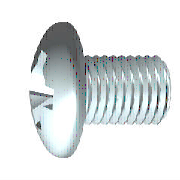
# Autodesk Inventor part: ISO 7045 - M4 x 6 - 4.8 - Z
Saved by Autodesk Inventor 2019.4 (Build 234330000, 330)
## iProperties
Created: 2018-01-05
Part Number: ISO 7045 - M4 x 6 - 4.8 - Z
Material: Stal
Description: Wkręt z łbem stożkowym ściętym z wgłębieniem krzyżowym w kształcie Z - Klasa dokładności A
Document SubType Name: Modeling
Standard: ISO 7045
Designer: barto
Standard Revision: Third edition 2011-09-01
Standards Organization: ISO
Language: pl-PL
Size Designation: M4 x 6 - 4.8 - Z
Categories: <MemberInstance><Categories><Category DisplayName="Mocowania" InternalName="e4da775c-781d-43d5-af7c-5136215cf5a6" Mnemonic="FSTN"><Category DisplayName="Śruby" InternalName="536e6df0-f778-49ac-b2f2-25c71d2aa0b2" Mnemonic="SCRW"><CategoryParameter DisplayName="Oznaczenie średnicy znamionowej" InternalName="03caf894-eafd-4c09-a035-916ac084b87b" Mnemonic="nomdiadesig"/><CategoryParameter DisplayName="Długość znamionowa" InternalName="238ecbaf-3e6c-45dd-aa95-4068c8e0fd02" Mnemonic="nomlen"/><CategoryParameter DisplayName="Oznaczenie gwintu" InternalName="586d5e89-370a-4089-914f-0110033585c7" Mnemonic="thrdesign"/><CategoryParameter DisplayName="Oznaczenie serii gwintów" InternalName="87c5849c-b3a5-4c3e-9c9b-2feecef9be86" Mnemonic="thrserdsgn"/><CategoryParameter DisplayName="Średnica znamionowa" InternalName="8bbe3f8e-44cf-40a9-a251-3a6edc8168d6" Mnemonic="nomdia"/><CategoryParameter DisplayName="Typ gwintu" InternalName="b4bbb7bc-d6aa-4c9f-a9a9-4152b9f6fe49" Mnemonic="thrtype"/><CategoryParameter DisplayName="Podziałka gwintu" InternalName="bb82302e-82d8-4176-8fc1-c5d7bb17d5ad" Mnemonic="pitch1"/><CategoryParameter DisplayName="Gwintów na jednostkę" InternalName="bdc6e7d2-ffd0-4d9c-a173-16b95ebb912d" Mnemonic="thrperunit1"/><CategoryParameter DisplayName="Klasa gwintu" InternalName="ebc0d23b-2cc6-4d2a-b376-d52aae53bab6" Mnemonic="thrclss"/><Category DisplayName="Z łbem okrągłym" InternalName="df3578aa-538f-4805-96a8-2439eb0c3cf7" Mnemonic="RNDSCRW"><CategoryParameter DisplayName="Długość uchwytu" InternalName="2c6ace26-543b-4217-91c4-9cdf8c3ec6f1" Mnemonic="grplen"/><CategoryParameter DisplayName="Wysokość łba" InternalName="2d152238-84fe-49ae-94c3-3fee884c292b" Mnemonic="headh"/><CategoryParameter DisplayName="Klasa właściwości" InternalName="85496db6-1567-48ed-b0d4-aa1f03366005" Mnemonic="propclss"/><CategoryParameter DisplayName="Długość gwintu" InternalName="a1e5edc5-4ca7-4847-8786-65b14d35af16" Mnemonic="thrlen"/><CategoryParameter DisplayName="Średnica trzonka" InternalName="c22f1a48-b8d5-43ef-ac5e-546ba91c0bd6" Mnemonic="grpdia"/><CategoryParameter DisplayName="Średnica łba" InternalName="e71ee7a1-06fd-425c-ba3b-09769885677c" Mnemonic="headdia"/></Category></Category></Category><Category DisplayName="TypDanych" InternalName="23b78d0f-2648-40c6-8793-ca6db495c9e8" Mnemonic="DATATYPE"><CategoryParameter DisplayName="NazwaWyświetlana" InternalName="05415f3d-3907-474b-a020-eb9d644f4cf3" Mnemonic="DISPLAYNAME"/><CategoryParameter DisplayName="Standardowe" InternalName="0c0a119c-1e12-4c84-803f-101930972f5e" Mnemonic="STANDARD"/><CategoryParameter DisplayName="Opis" InternalName="13903e3d-64b1-4950-80da-f627842ea37f" Mnemonic="DESCRIPTION"/><CategoryParameter DisplayName="Oznaczenie" InternalName="2675968c-4ce5-49e0-a4f5-552d29089031" Mnemonic="DESIGNATION"/><CategoryParameter DisplayName="Wiersz domyślny" InternalName="2af9ec52-faaa-4026-b378-f9fa4afca842" Mnemonic="DEFAULTROW"/><CategoryParameter DisplayName="Nazwa folderu" InternalName="3f06958e-8713-4116-9be7-ed6184ecc97b" Mnemonic="FOLDERNAME"/><CategoryParameter DisplayName="Wskazówki do poprawek" InternalName="45a75005-10b1-4dfc-8d6d-dfe629f0b93c" Mnemonic="REVISIONGUID"/><CategoryParameter DisplayName="Nazwa pliku" InternalName="8b46a4cc-9585-4fed-90c3-899f57e09a73" Mnemonic="FILENAME"/><CategoryParameter DisplayName="OrgStd" InternalName="8f5914e1-4693-403f-8ab5-d37768198c9d" Mnemonic="STDSORG"/><CategoryParameter DisplayName="Wersja rodziny" InternalName="914462f6-6e19-4b14-ba84-155b9680b1d0" Mnemonic="FAMILYREVISION"/><CategoryParameter DisplayName="Poprawka standardowa" InternalName="91d5a463-65c2-4fde-b823-3b7fea5e8e17" Mnemonic="STANDARDREVISION"/><CategoryParameter DisplayName="Zmiana elementu" InternalName="a65d44b9-392f-4f4f-857b-e4b3d54996fe" Mnemonic="MEMBERREVISION"/><CategoryParameter DisplayName="FormatKlipu" InternalName="bc51e27b-3422-4e78-93ef-cec197ddf230" Mnemonic="CLIPFORMAT"/><CategoryParameter DisplayName="Producent" InternalName="cd6c7a72-a28a-4e50-99a9-2c7f4e13e5ad" Mnemonic="MANUFACTURER"/><CategoryParameter DisplayName="NazwaWewnętrzna" InternalName="cf1d0246-76d9-4b4a-8305-fa0409afb5c1" Mnemonic="INTERNALNAME"/><CategoryParameter DisplayName="CzyMetryczne" InternalName="e2385c5b-1ea4-4823-96a8-8de651266ec3" Mnemonic="ISMETRIC"/><Category DisplayName="Część" InternalName="c0e0b642-3bcb-4cc8-9e80-f96d35c4afa4" Mnemonic="PART"><CategoryParameter DisplayName="Numer części" InternalName="016b6077-bfbe-49bd-92c9-d8d59c39c941" Mnemonic="PARTNUMBER"/><CategoryParameter DisplayName="Numer katalogowy" InternalName="4dba7c1c-e26c-444e-836c-b08b433409a8" Mnemonic="STOCKNUMBER"/><CategoryParameter DisplayName="Klucz - materiał" InternalName="5c9a8adb-dd2b-4535-b97f-0a94a95fe41f" Mnemonic="MATERIALKEY"/><CategoryParameter DisplayName="Materiał" InternalName="818a152a-d3c3-49ca-80ee-df7d91421b8e" Mnemonic="MATERIAL"/></Category></Category><Category DisplayName="Przekształcenie typowych DA" InternalName="924fff40-ddd0-4eff-ad42-30e3774ef79e" Mnemonic="LEGACYMAPDA"><CategoryParameter DisplayName="DACookie" InternalName="316934ee-8fe1-4c7a-9c36-f2d79e1add1a" Mnemonic="DACOOKIE"/></Category><Category DisplayName="MapaPowinowactwa" InternalName="cd87c42b-3e48-431e-b5c0-1cbeb14dfe77" Mnemonic="LEGACYMAP"><CategoryParameter DisplayName="niepowtarzalny ID elementu DA" InternalName="0918ad47-427f-4fed-ae26-24c81c58f590" Mnemonic="DACOOKIE"/><CategoryParameter DisplayName="ID Scalania11" InternalName="0ee8fb18-e2ed-4f39-96f6-1f4b5f50aa71" Mnemonic="MERGE11"/><CategoryParameter DisplayName="niepowtarzalny ID elementu CC" InternalName="5193edd4-b2b0-4ab4-9d54-de900eee34e0" Mnemonic="CCCOOKIE"/><CategoryParameter DisplayName="ID podziału" InternalName="72b5c83c-be7f-45c4-ae51-9160ea6deb26" Mnemonic="SPLIT"/><CategoryParameter DisplayName="IDczłonka" InternalName="8e5e0294-fc51-4c8f-b3d7-003dc5ed94f6" Mnemonic="MEMBERID"/><CategoryParameter DisplayName="NazwaKatalogu" InternalName="d99d1e27-aa94-4de2-af4c-c348882a6f4f" Mnemonic="CATALOGNAME"/><CategoryParameter DisplayName="NumerRodziny" InternalName="e705e1f4-09cb-413e-91f9-551b4188271e" Mnemonic="FAMILYNUMBER"/></Category></Categories><FamilyTemplate Id="si0152"><FamilyTemplateParameters><FamilyTemplateParameter ObjectType="kUserParameterObject" ValueType="xs:double" Id="1" ObjectReferenceKey="GUL"/><FamilyTemplateParameter ObjectType="kUserParameterObject" ValueType="xs:double" Id="2" ObjectReferenceKey="SPD"/><FamilyTemplateParameter ObjectType="kUserParameterObject" ValueType="xs:double" Id="3" ObjectReferenceKey="NLG"/><FamilyTemplateParameter ObjectType="kUserParameterObject" ValueType="xs:double" Id="4" ObjectReferenceKey="KOD"/><FamilyTemplateParameter ObjectType="kUserParameterObject" ValueType="xs:double" Id="5" ObjectReferenceKey="SBR"/><FamilyTemplateParameter ObjectType="kUserParameterObject" ValueType="xs:double" Id="6" ObjectReferenceKey="KR"/><FamilyTemplateParameter ObjectType="kUserParameterObject" ValueType="xs:double" Id="7" ObjectReferenceKey="PTC"/><FamilyTemplateParameter ObjectType="kUserParameterObject" ValueType="xs:double" Id="8" ObjectReferenceKey="GEL"/><FamilyTemplateParameter ObjectType="kUserParameterObject" ValueType="xs:double" Id="9" ObjectReferenceKey="THREADDIA"/><FamilyTemplateParameter ObjectType="kUserParameterObject" ValueType="xs:double" Id="10" ObjectReferenceKey="TOA"/><FamilyTemplateParameter ObjectType="kUserParameterObject" ValueType="xs:double" Id="11" ObjectReferenceKey="BDM"/><FamilyTemplateParameter ObjectType="kUserParameterObject" ValueType="xs:double" Id="12" ObjectReferenceKey="RR"/><FamilyTemplateParameter ObjectType="kUserParameterObject" ValueType="xs:double" Id="13" ObjectReferenceKey="STI"/><FamilyTemplateParameter ObjectType="kUserParameterObject" ValueType="xs:double" Id="14" ObjectReferenceKey="TPU"/><FamilyTemplateParameter ObjectType="kUserParameterObject" ValueType="xs:double" Id="15" ObjectReferenceKey="KOH"/><FamilyTemplateParameter ObjectType="kUserParameterObject" ValueType="xs:double" Id="16" ObjectReferenceKey="SDM"/><FamilyTemplateParameter ObjectType="kUserParameterObject" ValueType="xs:double" Id="17" ObjectReferenceKey="NND"/><FamilyTemplateParameter ObjectType="kUserParameterObject" ValueType="xs:double" Id="18" ObjectReferenceKey="GD"/><FamilyTemplateParameter ObjectType="kUserParameterObject" ValueType="xs:double" Id="19" ObjectReferenceKey="GAL"/><FamilyTemplateParameter ObjectType="kUserParameterObject" ValueType="xs:double" Id="20" ObjectReferenceKey="KEWI"/><FamilyTemplateParameter ObjectType="kUserParameterObject" ValueType="xs:double" Id="21" ObjectReferenceKey="GD1"/><FamilyTemplateParameter ObjectType="kPropertyObject" ValueType="xs:string" Id="100" ObjectReferenceKey="{32853F0F-3444-11d1-9E93-0060B03C1CA6}" SubObjectId="52"/><FamilyTemplateParameter ObjectType="kPropertyObject" ValueType="xs:string" Id="105" ObjectReferenceKey="{32853F0F-3444-11d1-9E93-0060B03C1CA6}" SubObjectId="5"/><FamilyTemplateParameter ObjectType="kPartComponentDefinitionObject" ValueType="xs:string" Id="110" SubObjectId="Material"/><FamilyTemplateParameter ObjectType="kThreadFeatureObject" ValueType="xs:structure" Id="300" ObjectReferenceKey="1002000010000000aa0f0000000000008000000000000000" SubObjectId="ThreadInfo"><FamilyTemplateParameter ObjectType="" ValueType="xs:string" Id="301" SubObjectId="ThreadDesignation"/><FamilyTemplateParameter ObjectType="" ValueType="xs:string" Id="302" SubObjectId="ThreadType"/><FamilyTemplateParameter ObjectType="" ValueType="xs:string" Id="303" SubObjectId="ThreadClass"/></FamilyTemplateParameter></FamilyTemplateParameters></FamilyTemplate><CategoryParameterMap><ParamToTemplateMap><ParamToTemplate CategoryParameter="//CategoryParameter[@InternalName='05415f3d-3907-474b-a020-eb9d644f4cf3']" ConstantValue="ISO 7045 Z"/><ParamToTemplate CategoryParameter="//CategoryParameter[@InternalName='cf1d0246-76d9-4b4a-8305-fa0409afb5c1']" ConstantValue="6647a0af-ffd5-424f-a826-2d82d1445c59"/><ParamToTemplate CategoryParameter="//CategoryParameter[@InternalName='3f06958e-8713-4116-9be7-ed6184ecc97b']" ConstantValue="ISO 7045  Z"/><ParamToTemplate CategoryParameter="//CategoryParameter[@InternalName='914462f6-6e19-4b14-ba84-155b9680b1d0']" ConstantValue="10"/><ParamToTemplate CategoryParameter="//CategoryParameter[@InternalName='bc51e27b-3422-4e78-93ef-cec197ddf230']" ConstantValue="CF_INVENTOR.STDPARTS"/><ParamToTemplate CategoryParameter="//CategoryParameter[@InternalName='e2385c5b-1ea4-4823-96a8-8de651266ec3']" ConstantValue="true"/><ParamToTemplate CategoryParameter="//CategoryParameter[@InternalName='13903e3d-64b1-4950-80da-f627842ea37f']" ConstantValue="Pan head screw with type Z cross recess - product grade A"/><ParamToTemplate CategoryParameter="//CategoryParameter[@InternalName='8f5914e1-4693-403f-8ab5-d37768198c9d']" ConstantValue="ISO"/><ParamToTemplate CategoryParameter="//CategoryParameter[@InternalName='0c0a119c-1e12-4c84-803f-101930972f5e']" ConstantValue="ISO 7045"/><ParamToTemplate CategoryParameter="//CategoryParameter[@InternalName='cd6c7a72-a28a-4e50-99a9-2c7f4e13e5ad']" TemplateParameter="104"/><ParamToTemplate CategoryParameter="//CategoryParameter[@InternalName='91d5a463-65c2-4fde-b823-3b7fea5e8e17']" ConstantValue="Third edition 2011-09-01"/><ParamToTemplate CategoryParameter="//CategoryParameter[@InternalName='45a75005-10b1-4dfc-8d6d-dfe629f0b93c']" ConstantValue="84d95e40-d300-4e1f-8614-c69d9a0839b2"/><ParamToTemplate CategoryParameter="//CategoryParameter[@InternalName='2af9ec52-faaa-4026-b378-f9fa4afca842']" ConstantValue="1"/><ParamToTemplate CategoryParameter="//CategoryParameter[@InternalName='d99d1e27-aa94-4de2-af4c-c348882a6f4f']" ConstantValue="ISO"/><ParamToTemplate CategoryParameter="//CategoryParameter[@InternalName='e705e1f4-09cb-413e-91f9-551b4188271e']" ConstantValue="15"/><ParamToTemplate CategoryParameter="//CategoryParameter[@InternalName='8b46a4cc-9585-4fed-90c3-899f57e09a73']" ConstantValue="ISO 7045 - M4 x 6 - 4.8 - Z - ISO"/><ParamToTemplate CategoryParameter="//CategoryParameter[@InternalName='a65d44b9-392f-4f4f-857b-e4b3d54996fe']" ConstantValue="496B91A0-027F-4D8C-B6E8-D4DF09B0C75A"/><ParamToTemplate CategoryParameter="//CategoryParameter[@InternalName='2c6ace26-543b-4217-91c4-9cdf8c3ec6f1']" ConstantValue="1,4"/><ParamToTemplate CategoryParameter="//CategoryParameter[@InternalName='ebc0d23b-2cc6-4d2a-b376-d52aae53bab6']" ConstantValue="6g"/><ParamToTemplate CategoryParameter="//CategoryParameter[@InternalName='03caf894-eafd-4c09-a035-916ac084b87b']" ConstantValue="M4"/><ParamToTemplate CategoryParameter="//CategoryParameter[@InternalName='b4bbb7bc-d6aa-4c9f-a9a9-4152b9f6fe49']" ConstantValue="ISO Metric profile"/><ParamToTemplate CategoryParameter="//CategoryParameter[@InternalName='8e5e0294-fc51-4c8f-b3d7-003dc5ed94f6']" ConstantValue="54"/><ParamToTemplate CategoryParameter="//CategoryParameter[@InternalName='316934ee-8fe1-4c7a-9c36-f2d79e1add1a']" ConstantValue="*Iso~I7045Z~M4x6 - 4.8 - Z~6*"/><ParamToTemplate CategoryParameter="//CategoryParameter[@InternalName='c22f1a48-b8d5-43ef-ac5e-546ba91c0bd6']" TemplateParameter="11"/><ParamToTemplate CategoryParameter="//CategoryParameter[@InternalName='2675968c-4ce5-49e0-a4f5-552d29089031']" TemplateParameter="100"/><ParamToTemplate CategoryParameter="//CategoryParameter[@InternalName='a1e5edc5-4ca7-4847-8786-65b14d35af16']" TemplateParameter="8"/><ParamToTemplate CategoryParameter="//CategoryParameter[@InternalName='e71ee7a1-06fd-425c-ba3b-09769885677c']" TemplateParameter="4"/><ParamToTemplate CategoryParameter="//CategoryParameter[@InternalName='2d152238-84fe-49ae-94c3-3fee884c292b']" TemplateParameter="15"/><ParamToTemplate CategoryParameter="//CategoryParameter[@InternalName='818a152a-d3c3-49ca-80ee-df7d91421b8e']" TemplateParameter="110"/><ParamToTemplate CategoryParameter="//CategoryParameter[@InternalName='238ecbaf-3e6c-45dd-aa95-4068c8e0fd02']" TemplateParameter="3"/><ParamToTemplate CategoryParameter="//CategoryParameter[@InternalName='8bbe3f8e-44cf-40a9-a251-3a6edc8168d6']" TemplateParameter="17"/><ParamToTemplate CategoryParameter="//CategoryParameter[@InternalName='016b6077-bfbe-49bd-92c9-d8d59c39c941']" TemplateParameter="105"/><ParamToTemplate CategoryParameter="//CategoryParameter[@InternalName='bb82302e-82d8-4176-8fc1-c5d7bb17d5ad']" TemplateParameter="7"/><ParamToTemplate CategoryParameter="//CategoryParameter[@InternalName='586d5e89-370a-4089-914f-0110033585c7']" TemplateParameter="301"/><ParamToTemplate CategoryParameter="//CategoryParameter[@InternalName='bdc6e7d2-ffd0-4d9c-a173-16b95ebb912d']" TemplateParameter="14"/></ParamToTemplateMap></CategoryParameterMap></MemberInstance>
Density: 7.85 g/cm^3
Appearance: Płyta
IsCustomPart: 0
Author: barto
Autodesk Inventor part; units mm, degrees
ref_plane "YZ Plane" through (0, 0, 0) normal (1, 0, 0) x (0, 1, 0)
ref_plane "XZ Plane" through (0, 0, 0) normal (0, 1, 0) x (-1, 0, 0)
ref_plane "XY Plane" through (0, 0, 0) normal (0, 0, 1) x (1, 0, 0)
sketch "Szkic1" plane through (0, 0, 0) normal (0, 0, 1) x (1, 0, 0)
  line L0 (6, 0) -> (6, 2)
  line L1 (6, 2) -> (1.4, 2)
  line L2 (3.9624, 5.08) -> (3.9624, 5.08)
  arc A0 (-1.7712, 3.9381) -> (-3.1, 0) centre (3.4, 0) ccw
  line L3 (-3.1, 0) -> (-3.1, 3.8917)
  line L4 (-2.7867, 1.9938) -> (-1.4714, 1.338)
  line L5 (-1.4714, 1.338) -> (-0.76, 0)
  line L6 (-0.76, 0) -> (6, 0)
  line L7 (-5.3079, 0) -> (7.8847, 0) projected
  line L8 (0, -1.016) -> (0, 6.096) projected
  line L9 (-2.7867, 1.9938) -> (-3.1, 2.15) construction
  line L10 (-1.7712, 3.9381) -> (-3.1, 3.8917)
  line L11 (-1.7712, 3.9381) -> (0, 4)
  line L12 (0, 4) -> (0, 1.8106)
  line L13 (0, 1.8106) -> (0.9706, 1.8106)
  line L14 (0.9706, 1.8106) -> (1.4, 2)
  line L15 (1.4, 2) -> (0, 2) construction
  dimension "d1" = 4
  dimension "d2" = 2.34
  dimension "d16" = 4.3
  dimension "d17" = 62
  dimension "d19" = 26.5
  dimension "d23" = 8
  dimension "d24" = 2
  dimension "d25" = 3.1
  dimension "d26" = 6.5
  dimension "d28" = 3.6211
  dimension "d29" = 4.6
  dimension "d30" = 0.4294
  dimension "d31" = 6
  constraints: 28 end point, 5 point on line, 4 collinear, 4 point on circle, 3 parallel, 2 perpendicular, 1 centre point, 1 horizontal, 1 tangent
  measures "d1" diameter of L1 L6
  measures "d2" distance from line of L5.end L3
  measures "d16" diameter of L9.end L6
  measures "d17" angle of L5 L6
  measures "d19" angle of L4 L6
  measures "d23" diameter of L11.end L6
  measures "d24" angle of L11 L6
  measures "d25" distance between parallel lines of L3 L12
  measures "d26" radius of A0
  measures "d28" diameter of L13 L6
  measures "d29" distance of L0.end L1.end
  measures "d30" horizontal distance of L13.end L1.end
  measures "d31" distance between parallel lines of L12 L0
revolve "Bryła" add sketch "Szkic1" angle 360 about axis through (-0.76, 0, 0) along (1, 0, 0) contours L6 L8 L13 L14 L1 L0 | L6 L5 L4 A0 L11 L8
ref_plane "Work Plane1" through (-3.1, 0, 0) normal (1, 0, 0) x (0, 1, 0)
sketch "Szkic2" plane through (-3.1, 0, 0) normal (1, 0, 0) x (0, 1, 0)
  circle A0 centre (0, 0) radius 3.9381 projected
  line L0 (-6.0699, 0) -> (8.8524, 0) projected
  line L1 (0, -6.0699) -> (0, 8.8524) projected
  line L2 (0, 2.15) -> (0, 0) construction
  line L3 (0, 0) -> (2.15, 0) construction
  arc A1 (0.86, 0) -> (0, 0.86) centre (0, 0) ccw construction
  line L4 (0, 0) -> (6.7207, 6.7207) construction
  line L5 (0.415, 2.1096) -> (0.2857, 1.0363)
  line L6 (2.1096, 0.415) -> (1.0363, 0.2857)
  arc A2 (0.2857, 1.0363) -> (0.7907, 0.7907) centre (0.5807, 1.0008) ccw
  arc A3 (0.7907, 0.7907) -> (1.0363, 0.2857) centre (1.0008, 0.5807) ccw
  arc A4 (2.15, 0) -> (2.1096, 0.415) centre (0, 0) ccw
  arc A5 (0.415, 2.1096) -> (0, 2.15) centre (0, 0) ccw
  arc A6 (2.1096, 0.415) -> (0.415, 2.1096) centre (0, 0) ccw
  line L7 (0.415, -2.1096) -> (0.2857, -1.0363)
  line L8 (2.1096, -0.415) -> (1.0363, -0.2857)
  arc A7 (0.7907, -0.7907) -> (0.2857, -1.0363) centre (0.5807, -1.0008) ccw
  arc A8 (1.0363, -0.2857) -> (0.7907, -0.7907) centre (1.0008, -0.5807) ccw
  arc A9 (2.1096, -0.415) -> (2.15, 0) centre (0, 0) ccw
  arc A10 (0, -2.15) -> (0.415, -2.1096) centre (0, 0) ccw
  arc A11 (0.415, -2.1096) -> (2.1096, -0.415) centre (0, 0) ccw
  line L9 (-0.415, 2.1096) -> (-0.2857, 1.0363)
  line L10 (-2.1096, 0.415) -> (-1.0363, 0.2857)
  arc A12 (-0.7907, 0.7907) -> (-0.2857, 1.0363) centre (-0.5807, 1.0008) ccw
  arc A13 (-1.0363, 0.2857) -> (-0.7907, 0.7907) centre (-1.0008, 0.5807) ccw
  arc A14 (-2.1096, 0.415) -> (-2.15, 0) centre (0, 0) ccw
  arc A15 (0, 2.15) -> (-0.415, 2.1096) centre (0, 0) ccw
  arc A16 (-0.415, 2.1096) -> (-2.1096, 0.415) centre (0, 0) ccw
  arc A17 (-0.415, -2.1096) -> (0, -2.15) centre (0, 0) ccw
  arc A18 (-2.1096, -0.415) -> (-0.415, -2.1096) centre (0, 0) ccw
  arc A19 (-2.15, 0) -> (-2.1096, -0.415) centre (0, 0) ccw
  line L11 (-2.1096, -0.415) -> (-1.0363, -0.2857)
  line L12 (-0.415, -2.1096) -> (-0.2857, -1.0363)
  arc A20 (-0.2857, -1.0363) -> (-0.7907, -0.7907) centre (-0.5807, -1.0008) ccw
  arc A21 (-0.7907, -0.7907) -> (-1.0363, -0.2857) centre (-1.0008, -0.5807) ccw
  arc A22 (1.075, 0) -> (0, 1.075) centre (0, 0) ccw construction
  dimension "d4" = 45
  dimension "d5" = 1.72
  dimension "d6" = 4.3
  dimension "d7" = 0.415
  dimension "d20" = 2.15
  constraints: 46 point on circle, 25 symmetric about line, 22 centre point, 22 end point, 6 tangent, 4 coincident, 3 collinear, 3 point on line, 1 midpoint, 1 perpendicular, 22 other
  measures "d4" angle of L4 L3
  measures "d5" diameter of A1
  measures "d6" diameter of A6
  measures "d7" distance from line of L5.start L2
  measures "d20" diameter of A22
extrude "Szczelina" add sketch "Szkic2" along normal up to next draft 5 contours L6 A3 A2 L5 A6 | A11 L7 A7 A8 L8 | L9 A12 A13 L10 A16 | A18 L11 A21 A20 L12
revolve "Wycięcie" cut sketch "Szkic1" angle 360 about axis through (-10, 0, 0) along (1, 0, 0) contours L3 L10 A0
sketch "Szkic4" plane through (-3.1, 0, 0) normal (1, 0, 0) x (0, 1, 0)
  circle A0 centre (0, 0) radius 3.9381 projected
  line L0 (-8.9998, 0) -> (8.9998, 0) projected
  line L1 (0, -8.9998) -> (0, 8.9998) projected
  line L2 (0, 0) -> (6.4284, 6.4284) construction
  circle A1 centre (0, 0) radius 0.2075 construction
  line L3 (0, 0) -> (6.4284, -6.4284) construction
  line L4 (0, 0) -> (-6.4284, 6.4284) construction
  line L5 (0, 0) -> (-6.4284, -6.4284) construction
  line L6 (1.5203, 1.5203) -> (0, 0.2075)
  line L7 (-1.5203, 1.5203) -> (-0.2075, 0)
  line L8 (-1.5203, -1.5203) -> (0, -0.2075)
  line L9 (1.5203, -1.5203) -> (0.2075, 0)
  line L10 (1.5203, 1.5203) -> (0.2075, 0)
  line L11 (-1.5203, 1.5203) -> (0, 0.2075)
  line L12 (-1.5203, -1.5203) -> (-0.2075, 0)
  line L13 (1.5203, -1.5203) -> (0, -0.2075)
  circle A2 centre (0, 0) radius 2.15 construction
  dimension "d11" = 0.415
  dimension "d14" = 45
  dimension "d35" = 1.5203
  constraints: 24 end point, 10 point on line, 7 point on circle, 3 perpendicular, 3 symmetric about line, 2 centre point, 2 coincident, 3 other
  measures "d11" diameter of A1
  measures "d14" angle of L2 L0
  measures "d35" distance from line of L0 L6.start
extrude "Wycięcie o kształcie gwiazdy" cut sketch "Szkic4" along normal blind 3.1 draft -10 contours L9 L13 L1 L0 | L0 L1 L6 L10 | L1 L0 L7 L11 | L8 L12 L0 L1
fillet "Zaokrąglenie1" radius 1.3 1 edges at (-1.7712, -3.9381, 0)
fillet "Zaokrąglenie2" radius 0.166 5 edges at (-2.7867, 0, 1.9938) (-2.7867, -1.9938, 0) (-2.7867, 0, -1.9938) (-2.7867, 1.9851, 0.1854) (-2.7867, 1.9851, -0.1854)
thread "Gwint" size "M4x0.7" class "6g" standard "ISO Metric profile" length 4.6
chamfer "Faza1" distance 0.4294 distance2 0.4295 1 edges at (6, -2, 0) measured on face at (6, -1.5, 0)
ref_plane "Work Plane3" through (1.85, 0, 0) normal (0, 1, 0) x (1, 0, 0)
equation "\"d11\" = 0.5 * SBR"
equation "\"d35\" = 0.353553 * SDM"
equation "\"d12\" = KOH"
equation "\"d5\" = 0.4 * SDM"
equation "\"d6\" = SDM"
equation "\"d7\" = 0.5 * SBR"
equation "\"d20\" = 0.5 * SDM"
equation "\"d1\" = GD"
equation "\"d2\" = STI"
equation "\"d16\" = SDM"
equation "\"d23\" = KOD"
equation "\"d24\" = KEWI"
equation "\"d25\" = KOH"
equation "\"d26\" = KR"
equation "\"d28\" = BDM"
equation "\"d29\" = GEL"
equation "\"d30\" = GAL"
equation "\"d31\" = NLG"
equation "\"d32\" = RR"
equation "\"d22\" = 0.2 * SBR"
equation "\"d8\" = GEL"
equation "\"d36\" = -0.5 * SPD + 0.5 * GD"
equation "\"GD\" = 4"
equation "\"NLG\" = 6"
equation "\"GEL\" = 4.6"
equation "\"KOD\" = 8"
equation "\"KOH\" = 3.1"
equation "\"SDM\" = 4.3"
equation "\"STI\" = 2.34"
equation "\"SBR\" = 0.83"
equation "\"KEWI\" = 2deg"
equation "\"d3\" = -KOH"
equation "\"KR\" = 6.5"
equation "\"BDM\" = 3.62111"
equation "\"GAL\" = 0.61345 * PTC"
equation "\"GUL\" = 0.61345 * PTC"
equation "\"RR\" = 1.3"
equation "\"SPD\" = NND - 1.2269 * PTC"
equation "\"PTC\" = 0.7"
equation "\"THREADDIA\" = 4"
equation "\"TOA\" = 30deg"
equation "\"NND\" = 4"
equation "\"GD1\" = THREADDIA - 1.2269 * PTC"
body "Solid1"
